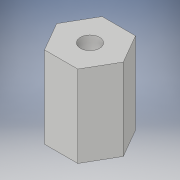
# Autodesk Inventor part: Pololu Hex Wheel Adapter 4mm
Saved by Autodesk Inventor 2018.3 (Build 223284000, 284)
## iProperties
Created: 2018-08-03
Part Number: Pololu Hex Wheel Adapter 4mm
Material: Generisch
Document SubType Name: Modeling
Designer: JochenAlt
Density: 1 g/cm^3
Appearance: Vorgabe
Author: JochenAlt
Autodesk Inventor part; units mm, degrees
ref_plane "YZ Plane" through (0, 0, 0) normal (1, 0, 0) x (0, 1, 0)
ref_plane "XZ Plane" through (0, 0, 0) normal (0, 1, 0) x (-1, 0, 0)
ref_plane "XY Plane" through (0, 0, 0) normal (0, 0, 1) x (1, 0, 0)
sketch "Skizze1" plane through (0, 0, 0) normal (0, 0, 1) x (1, 0, 0)
  circle A0 centre (0, 0) radius 6 construction
  line L0 (3.4641, 6) -> (6.9282, 0)
  line L1 (6.9282, 0) -> (3.4641, -6)
  line L2 (3.4641, -6) -> (-3.4641, -6)
  line L3 (-3.4641, -6) -> (-6.9282, 0)
  line L4 (-6.9282, 0) -> (-3.4641, 6)
  line L5 (-3.4641, 6) -> (3.4641, 6)
  circle A1 centre (0, 0) radius 2
  point P0 (0, 6)
  dimension "d0" = 12
  dimension "d1" = 4
  constraints: 12 end point, 3 coincident, 1 centre point, 1 midpoint, 1 vertical alignment, 15 other
  measures "d1" diameter of A1
extrude "Extrusion1" add sketch "Skizze1" along normal blind 17
